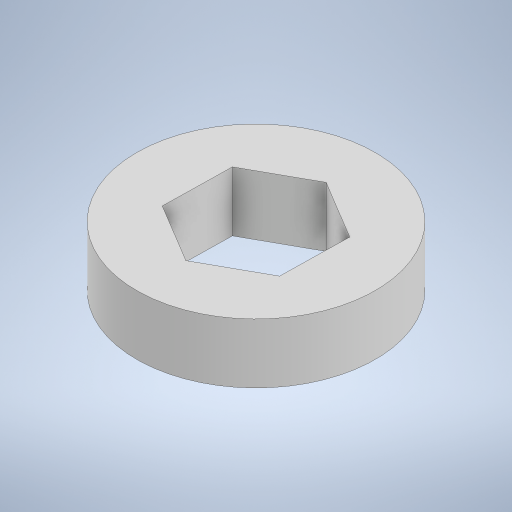
# Autodesk Inventor part: 4-bar intake spacer
Saved by Autodesk Inventor 2023 (Build 270158030, 158C)
## iProperties
Created: 2022-07-19
Part Number: 4-bar intake spacer
Material: Generic
Document SubType Name: Modeling
Designer: rm0990889
Density: 1 g/cm^3
Appearance: Default
Author: rm0990889
Autodesk Inventor part; units mm, degrees
ref_plane "YZ Plane" through (0, 0, 0) normal (1, 0, 0) x (0, 1, 0)
ref_plane "XZ Plane" through (0, 0, 0) normal (0, 1, 0) x (-1, 0, 0)
ref_plane "XY Plane" through (0, 0, 0) normal (0, 0, 1) x (1, 0, 0)
sketch "Sketch1" plane through (0, 0, 0) normal (0, 1, 0) x (-1, 0, 0)
  circle A0 centre (0, 0) radius 6.35
  line L0 (-0.1298, -7.3312) -> (-6.4139, -3.5532)
  line L1 (-6.4139, -3.5532) -> (-6.2841, 3.778)
  line L2 (-6.2841, 3.778) -> (0.1298, 7.3312)
  line L3 (0.1298, 7.3312) -> (6.4139, 3.5532)
  line L4 (6.4139, 3.5532) -> (6.2841, -3.778)
  line L5 (6.2841, -3.778) -> (-0.1298, -7.3312)
  circle A1 centre (0, 0) radius 12.7
  point P0 (3.0772, -5.5546)
  dimension "d0" = 12.7
  dimension "d1" = 25.4
  constraints: 12 end point, 3 coincident, 1 centre point, 1 midpoint, 16 other
  measures "d1" diameter of A1
extrude "Extrusion1" add sketch "Sketch1" along normal blind 6.35
body "Solid1"
